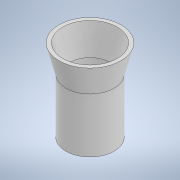
# Autodesk Inventor part: 20mm Nozzle
Saved by Autodesk Inventor 2022 (Build 260153000, 153)
## iProperties
Created: 2023-01-19
Part Number: 20mm Nozzle
Material: Generic
Document SubType Name: Modeling
Designer: ASUS
Density: 1 g/cm^3
Appearance: Default
Author: ASUS
Autodesk Inventor part; units mm, degrees
ref_plane "YZ Plane" through (0, 0, 0) normal (1, 0, 0) x (0, 1, 0)
ref_plane "XZ Plane" through (0, 0, 0) normal (0, 1, 0) x (-1, 0, 0)
ref_plane "XY Plane" through (0, 0, 0) normal (0, 0, 1) x (1, 0, 0)
sketch "Sketch1" plane through (0, 0, 0) normal (0, 1, 0) x (-1, 0, 0)
  circle A0 centre (0, 0) radius 7.5
  circle A1 centre (0, 0) radius 8.875
  dimension "d0" = 15
  dimension "d1" = 17.75
  constraints: 2 centre point, 2 coincident
  measures "d0" diameter of A0
  measures "d1" diameter of A1
extrude "Extrusion1" add sketch "Sketch1" along normal blind 20
sketch "Sketch2" plane through (0, 0, 0) normal (1, 0, 0) x (0, 1, 0)
  line L0 (30, 0) -> (30, -10) construction
  line L1 (20, -8.875) -> (20, 8.875) projected
  line L2 (20, -7.5) -> (0, -7.5) projected
  line L3 (20, -7.5) -> (30, -10)
  line L4 (20, -8.875) -> (30, -11.375)
  line L5 (30, -11.375) -> (30, -10)
  line L6 (20, 0) -> (30, 0)
  point P0 (0, 0)
  dimension "d4" = 10
  dimension "d5" = 10
  constraints: 10 end point, 2 point on line, 1 midpoint, 1 parallel, 1 perpendicular, 1 vertical
  measures "d4" distance between parallel lines of L1 L0
  measures "d5" distance of L0.start L0.end
revolve "Revolution1" add sketch "Sketch2" angle 360 about axis through (0, 20, 0) along (0, 1, 0)
body "Solid1"
